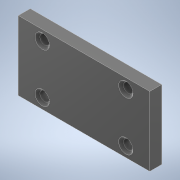
# Autodesk Inventor part: Tampa Apoio Motor
Saved by Autodesk Inventor 2021 (Build 250183000, 183)
## iProperties
Created: 2022-11-17
Part Number: Tampa Apoio Motor
Material: Plástico PC/ABS
Document SubType Name: Modeling
Designer: nicho
Density: 0.357273 g/cm^3
Appearance: Liso - Preto
Mass: 2.84925 g
Surface Area: 40.3 cm^2
Volume: 7.975 cm^3
Author: nicho
Autodesk Inventor part; units mm, degrees
ref_plane "YZ Plane" through (0, 0, 0) normal (1, 0, 0) x (0, 1, 0)
ref_plane "XZ Plane" through (0, 0, 0) normal (0, 1, 0) x (-1, 0, 0)
ref_plane "XY Plane" through (0, 0, 0) normal (0, 0, 1) x (1, 0, 0)
sketch "Esboço1" plane through (0, 0, 0) normal (0, 0, 1) x (1, 0, 0)
  line L0 (27.5, -14.5) -> (-27.5, -14.5)
  line L1 (-27.5, -14.5) -> (-27.5, 14.5)
  line L2 (-27.5, 14.5) -> (27.5, 14.5)
  line L3 (27.5, 14.5) -> (27.5, -14.5)
  line L4 (27.5, -14.5) -> (-27.5, 14.5) construction
  line L5 (-27.5, -14.5) -> (27.5, 14.5) construction
  point P0 (0, 0)
  dimension "d0" = 55
  dimension "d1" = 29
  constraints: 12 end point, 2 midpoint, 2 parallel, 1 horizontal, 1 perpendicular
  measures "d0" distance of L1.end L2.end
  measures "d1" distance of L0.end L1.end
extrude "Extrusão1" add sketch "Esboço1" along normal blind 5
sketch "Esboço2" plane through (0, 0, 5) normal (0, 0, 1) x (1, 0, 0)
  line L0 (-27.5, 14.5) -> (-27.5, -14.5) projected
  line L1 (27.5, 14.5) -> (-27.5, 14.5) projected
  line L2 (0, 0) -> (-7.3879, 0)
  line L3 (0, 0) -> (0, 5.1516)
  point P0 (-17.5, 10.25)
  point P1 (17.5, 10.25)
  point P2 (-17.5, -10.25)
  point P3 (17.5, -10.25)
  dimension "d4" = 10
  dimension "d5" = 4.25
  constraints: 4 end point, 3 symmetric about line, 1 horizontal, 1 vertical
  measures "d4" distance from line of L0 point (-17.5, 10.25)
  measures "d5" distance from line of L1 point (-17.5, 10.25)
hole "Furo1" at (-17.5, 10.25, 5) at (17.5, 10.25, 5) at (-17.5, -10.25, 5) at (17.5, -10.25, 5) direction (0, 0, -1) diameter 4 end through all countersink diameter 6 countersink angle 90
